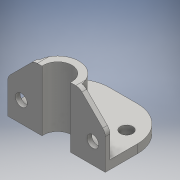
# Autodesk Inventor part: 240516_3Dsketch02
Saved by Autodesk Inventor 2016 (Build 200138000, 138)
## iProperties
Created: 2024-05-16
Part Number: 240516_3Dsketch02
Material: 일반
Document SubType Name: Modeling
Designer: pc
Density: 1 g/cm^3
Appearance: 기본값
Author: pc
Autodesk Inventor part; units mm, degrees
ref_plane "YZ Plane" through (0, 0, 0) normal (1, 0, 0) x (0, 1, 0)
ref_plane "XZ Plane" through (0, 0, 0) normal (0, 1, 0) x (-1, 0, 0)
ref_plane "XY Plane" through (0, 0, 0) normal (0, 0, 1) x (1, 0, 0)
sketch "스케치1" plane through (0, 0, 0) normal (0, 0, 1) x (1, 0, 0)
  line L0 (28.2247, -19.3821) -> (-28.2247, -19.3821)
  line L1 (-28.2247, -19.3821) -> (-28.2247, 19.3821)
  line L2 (-28.2247, 19.3821) -> (28.2247, 19.3821)
  line L3 (28.2247, 19.3821) -> (28.2247, -19.3821)
  line L4 (28.2247, -19.3821) -> (-28.2247, 19.3821) construction
  line L5 (-28.2247, -19.3821) -> (28.2247, 19.3821) construction
  point P0 (0, 0)
  constraints: 12 end point, 2 midpoint, 2 parallel, 1 horizontal, 1 perpendicular
extrude "돌출1" add sketch "스케치1" along normal blind 35
sketch "스케치2" plane through (0, 0, 35) normal (0, 0, 1) x (1, 0, 0)
  line L0 (-28.2247, -19.3821) -> (28.2247, -19.3821) projected
  arc A0 (8.0086, -19.3821) -> (-8.4193, -19.3821) centre (-0.2053, -18.5165) ccw
  arc A1 (12.0005, -16.6695) -> (-12.4112, -16.6695) centre (-0.2053, -18.5165) ccw
  line L1 (28.2247, -19.3821) -> (28.2247, 19.3821) projected
  line L2 (28.2247, -16.6695) -> (12.0005, -16.6695)
  line L3 (-12.4112, -16.6695) -> (-28.2247, -16.6695)
  line L4 (28.2247, -16.6695) -> (28.2247, 19.3821)
  line L5 (28.2247, 19.3821) -> (-28.2247, 19.3821) projected
  line L6 (-28.2247, 19.3821) -> (-28.2247, -16.6695)
  point P0 (0, 0)
  constraints: 8 end point, 5 point on line, 4 point on circle, 2 centre point, 2 perpendicular, 1 vertical
extrude "돌출2" cut sketch "스케치2" against normal blind 30 contours L2 A1 L3 L6 L5 L1
extrude "돌출3" cut sketch "스케치2" against normal blind 35 contours A0 L0
sketch "스케치3" plane through (-28.2247, -16.6695, 35) normal (0, 1, 0) x (1, 0, 0)
  circle A0 centre (7.8268, 23.0556) radius 3.4368
  circle A1 centre (49.2387, 23.0556) radius 3.3984
  point P0 (28.2247, 35)
  constraints: 2 centre point
extrude "돌출4" cut sketch "스케치3" against normal blind 35
chamfer "모따기1" distance 15 angle 45 1 edges at (-28.2247, -18.0258, 35)
chamfer "모따기2" distance 15 angle 45 1 edges at (28.2247, -18.0258, 35)
fillet "모깎기1" radius 5 4 edges at (28.2247, -18.0258, 20) (13.2247, -18.0258, 35) (-13.2247, -18.0258, 35) (-28.2247, -18.0258, 20)
sketch "스케치4" plane through (0, 0, 5) normal (0, 0, 1) x (1, 0, 0)
  circle A0 centre (18.185, 3.0025) radius 3.5989
  circle A1 centre (-16.9318, 3.0025) radius 3.8942
  line L0 (-28.2247, 19.3821) -> (28.2247, 19.3821) projected
  arc A2 (-10.8118, 19.3821) -> (-28.2247, -16.6695) centre (16.7776, -16.1746) ccw
  line L1 (28.2247, 19.3821) -> (28.2247, -19.3821) projected
  arc A3 (28.2247, -16.6695) -> (8.7119, 19.3821) centre (-7.9765, -12.9568) ccw
  line L2 (-28.2247, -16.6695) -> (-28.2247, 19.3821) projected
  line L3 (-28.2247, -16.6695) -> (-28.2247, 19.3821)
  line L4 (-28.2247, 19.3821) -> (-10.8118, 19.3821)
  line L5 (8.7119, 19.3821) -> (28.2247, 19.3821)
  point P0 (0, 0)
  constraints: 6 end point, 4 centre point, 4 point on circle, 3 collinear, 3 point on line
extrude "돌출5" cut sketch "스케치4" against normal blind 35 contours A0 | A1
sketch "스케치5" plane through (0, 0, 0) normal (0, 0, -1) x (-1, 0, 0)
  point P0 (0, 0)
fillet "모깎기2" radius 20 2 edges at (28.2247, 19.3821, 2.5) (-28.2247, 19.3821, 2.5)
